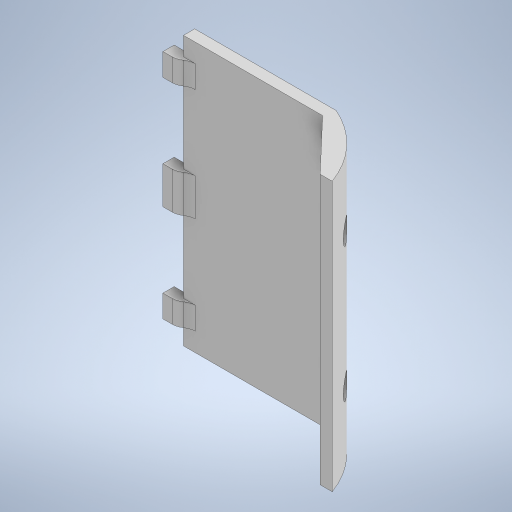
# Autodesk Inventor part: pokrywka_baterii
Saved by Autodesk Inventor 2023 (Build 270158000, 158)
## iProperties
Created: 2024-04-25
Part Number: pokrywka_baterii
Material: Ogólny
Document SubType Name: Modeling
Designer: Kamil
Density: 1 g/cm^3
Appearance: Domyślna
Author: Kamil
Autodesk Inventor part; units mm, degrees
ref_plane "YZ Plane" through (0, 0, 0) normal (1, 0, 0) x (0, 1, 0)
ref_plane "XZ Plane" through (0, 0, 0) normal (0, 1, 0) x (-1, 0, 0)
ref_plane "XY Plane" through (0, 0, 0) normal (0, 0, 1) x (1, 0, 0)
sketch "Szkic1" plane through (0, 0, 0) normal (0, 1, 0) x (-1, 0, 0)
  arc A0 (-57.7209, 16.9104) -> (-41.8849, 0) centre (-30, 27) ccw
  line L0 (-41.8849, 0) -> (-4, 0)
  line L1 (-4, 0) -> (-4, 3)
  line L2 (-57.7209, 16.9104) -> (-54.5041, 16.9104)
  line L3 (-54.5041, 16.9104) -> (-41.2361, 3)
  line L4 (-41.2361, 3) -> (-4, 3)
  line L5 (-4, 1.5) -> (-4, 3)
  dimension "d3" = 27
  dimension "d4" = 29.5
  dimension "d8" = 37.8849
  dimension "d9" = 37.2361
  dimension "d10" = 19.2234
  constraints: 12 end point, 2 horizontal, 2 point on circle, 1 centre point
  measures "d3" distance from line of L0 A0.centre
  measures "d4" radius of A0
  measures "d8" distance of L0.end L0.start
  measures "d9" distance of L3.end L1.end
  measures "d10" distance of L2.end L3.end
extrude "Wyciągnięcie proste1" add sketch "Szkic1" along normal blind 72
sketch "Szkic3" plane through (4, 0, 0) normal (-1, 0, 0) x (0, 0, 1)
  line L0 (0, 0) -> (3, 0) projected
  line L1 (3, 0) -> (3, 72) projected
  line L2 (0, 72) -> (3, 72) projected
  line L3 (0, 0) -> (0, 72) projected
  line L4 (1.5, 5) -> (4.5, 5)
  line L5 (4.5, 5) -> (4.5, 11)
  line L6 (4.5, 11) -> (1.5, 11)
  line L7 (1.5, 11) -> (1.5, 5)
  line L8 (0, 0) -> (0, 72) projected
  line L9 (0, 36) -> (-11, 36)
  line L10 (1.5, 31) -> (4.5, 31)
  line L11 (4.5, 31) -> (4.5, 41)
  line L12 (4.5, 41) -> (1.5, 41)
  line L13 (1.5, 41) -> (1.5, 31)
  line L14 (1.5, 67) -> (4.5, 67)
  line L15 (4.5, 67) -> (4.5, 61)
  line L16 (4.5, 61) -> (1.5, 61)
  line L17 (1.5, 61) -> (1.5, 67)
  point P0 (1.5, 36)
  point P1 (0, 36)
  dimension "d15" = 3
  dimension "d16" = 6
  dimension "d17" = 4.5
  dimension "d18" = 5
  dimension "d19" = 3
  dimension "d20" = 10
  dimension "d21" = 4.5
  constraints: 26 end point, 4 parallel, 4 symmetric about line, 3 horizontal, 3 midpoint, 2 perpendicular, 1 horizontal alignment
  measures "d15" distance of L6.end L5.end
  measures "d16" distance of L5.end L4.end
  measures "d17" distance between parallel lines of L3 L5
  measures "d18" distance between parallel lines of L4 L0
  measures "d19" distance of L12.end L11.end
  measures "d20" distance of L11.end L10.end
  measures "d21" distance between parallel lines of L11 L3
extrude "Wyciągnięcie proste2" add sketch "Szkic3" along normal blind 4 contours L4 L7 L6 L1 | L1 L6 L5 L4 | L10 L13 L12 L1 | L1 L12 L11 L10 | L14 L15 L16 L1 | L1 L16 L17 L14
fillet "Zaokrąglenie1" radius 4 6 edges at (4, 8, 3) (4, 36, 3) (4, 64, 3) (4, 36, 4.5) (4, 8, 4.5) (4, 64, 4.5)
fillet "Zaokrąglenie2" radius 1 3 edges at (4, 64, 1.5) (4, 36, 1.5) (4, 8, 1.5)
sketch "Szkic4" plane through (54.5041, 0, 16.9104) normal (-0.7236188, 0, 0.6901999) x (0.6901999, 0, 0.7236188)
  line L0 (-19.2234, 0) -> (0, 0) projected
  line L1 (0, 0) -> (0, 72) projected
  line L2 (-19.2234, 72) -> (0, 72) projected
  line L3 (-19.2234, 0) -> (-19.2234, 72) projected
  line L4 (-19.2234, 36) -> (0, 36)
  circle A0 centre (-7, 18) radius 1.6
  circle A1 centre (-7, 54) radius 1.6
  point P0 (-49.8554, 0)
  point P1 (-9.6117, 36)
  dimension "d26" = 3.2
  dimension "d27" = 36
  dimension "d34" = 7
  constraints: 3 midpoint, 2 centre point, 2 end point, 1 other
  measures "d26" diameter of A0
  measures "d27" diameter of A0.centre L4
  measures "d34" distance from line of L1 A0.centre
extrude "Wyciągnięcie proste3" cut sketch "Szkic4" against normal through all contours A0 | A1
ref_plane "Płaszczyzna konstrukcyjna1" through (51.3468, 0, 6.6391) normal (-0.7236188, 0, 0.6901999) x (0.6901999, 0, 0.7236188)
sketch "Szkic5" plane through (51.3468, 0, 6.6391) normal (-0.7236188, 0, 0.6901999) x (0.6901999, 0, 0.7236188)
  circle A0 centre (2.6117, 54) radius 1.6 projected
  circle A1 centre (2.6117, 18) radius 1.6 projected
  line L0 (-9.6117, 0) -> (9.6117, 0) projected
  line L1 (9.6117, 0) -> (9.6117, 72) projected
  line L2 (-9.6117, 72) -> (9.6117, 72) projected
  line L3 (-9.6117, 0) -> (-9.6117, 72) projected
  circle A2 centre (2.6117, 54) radius 1.6 projected
  circle A3 centre (2.6117, 54) radius 3
  circle A4 centre (2.6117, 18) radius 1.6 projected
  circle A5 centre (2.6117, 18) radius 3
  point P0 (-40.2437, 0)
  dimension "d30" = 6
  dimension "d31" = 6
  constraints: 2 centre point, 2 coincident
  measures "d30" diameter of A3
  measures "d31" diameter of A5
extrude "Wyciągnięcie proste4" cut sketch "Szkic5" along normal blind 3.3 contours A0 | A1 | A3 | A5
